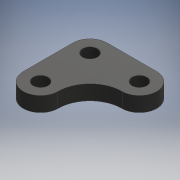
# Autodesk Inventor part: Updown_triangle
Saved by Autodesk Inventor 2016 (Build 200138000, 138)
## iProperties
Created: 2015-12-07
Part Number: Updown_triangle
Material: Generic
Document SubType Name: Modeling
Designer: lk8187
Density: 1 g/cm^3
Appearance: Smooth - Dark Gray
Author: lk8187
Autodesk Inventor part; units mm, degrees
ref_plane "YZ Plane" through (0, 0, 0) normal (1, 0, 0) x (0, 1, 0)
ref_plane "XZ Plane" through (0, 0, 0) normal (0, 1, 0) x (-1, 0, 0)
ref_plane "XY Plane" through (0, 0, 0) normal (0, 0, 1) x (1, 0, 0)
sketch "Sketch1" plane through (0, 0, 0) normal (0, 0, 1) x (1, 0, 0)
  line L0 (10, 0) -> (0, 0) construction
  line L1 (0, 0) -> (0, -10) construction
  line L2 (0, 3.5) -> (10, 3.5)
  arc A0 (10, -3.5) -> (10, 3.5) centre (10, 0) ccw
  arc A1 (0, 3.5) -> (-3.5, 0) centre (0, 0) ccw
  line L3 (-3.5, 0) -> (-3.5, -10)
  arc A2 (-3.5, -10) -> (3.5, -10) centre (0, -10) ccw
  arc A3 (10, -3.5) -> (3.5, -10) centre (10, -10) ccw
  line L4 (3.5, -10) -> (3.5, -3.5) construction
  line L5 (3.5, -3.5) -> (10, -3.5) construction
  dimension "d0" = 10
  dimension "d2" = 3.5
  constraints: 12 end point, 9 point on circle, 9 tangent, 6 coincident, 4 centre point, 3 horizontal, 2 vertical, 1 perpendicular
  measures "d0" distance of L0.start L0.end
  measures "d2" radius of A0
extrude "Extrusion1" add sketch "Sketch1" against normal blind 3
hole "Hole1" at (0, 0, 0) at (0, -10, 0) at (10, 0, 0) direction (0, 0, -1) diameter 3 depth 8 tip angle 118
body "Solid1"
